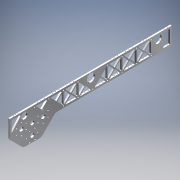
# Autodesk Inventor part: Inner Plate
Saved by Autodesk Inventor 2019.4 (Build 234330000, 330)
## iProperties
Created: 2019-12-07
Part Number: Inner Plate
Material: Aluminum 6061
Document SubType Name: Modeling
Designer: admin
Density: 2.7 g/cm^3
Appearance: Aluminum - Flat
Mass: 787.136 g
Surface Area: 1230.91 cm^2
Volume: 291.532 cm^3
Author: admin
Autodesk Inventor part; units mm, degrees
ref_plane "YZ Plane" through (0, 0, 0) normal (1, 0, 0) x (0, 1, 0)
sketch "Sketch1" plane through (0, 0, 0) normal (1, 0, 0) x (0, 1, 0)
  line L0 (80, -100) -> (0, -100)
  line L1 (0, -100) -> (0, 100)
  line L2 (0, 100) -> (80, 100)
  line L3 (80, 100) -> (80, -100)
  line L4 (30, -90) -> (30, 90) construction
  line L5 (30, 0) -> (95.4693, 0) construction
  line L6 (60, -40) -> (-60, -40) construction
  line L7 (-60, -40) -> (-60, 40)
  line L8 (-60, 40) -> (60, 40) construction
  line L9 (60, 40) -> (60, -40) construction
  line L10 (60, -40) -> (-60, 40) construction
  line L11 (-60, -40) -> (60, 40) construction
  line L12 (-60, -40) -> (0, -100)
  line L13 (-60, -40) -> (24.8528, -40) construction
  line L14 (-60, 40) -> (0, 100)
  point P0 (0, 0)
  point P1 (0, 0)
  point P2 (0, 0)
  dimension "d2" = 80
  dimension "d3" = 200
  dimension "d7" = 180
  dimension "d8" = 30
  dimension "d9" = 100
  dimension "d10" = 120
  dimension "d11" = 80
  dimension "d12" = 45
  dimension "d13" = 45
  constraints: 30 end point, 5 midpoint, 4 horizontal, 4 parallel, 2 perpendicular, 2 point on line, 1 coincident, 1 equal length, 1 vertical
  measures "d2" distance of L0.start L0.end
  measures "d3" distance of L2.end L0.start
  measures "d7" distance of L4.end L4.start
  measures "d8" distance between parallel lines of L1 L4
  measures "d9" distance between parallel lines of L0 L5
  measures "d10" distance of L7.end L8.end
  measures "d11" distance of L6.end L7.end
  measures "d12" angle of L12 L13
  measures "d13" angle of L8 L14
extrude "Extrusion1" add sketch "Sketch1" along normal blind 7
sketch "Sketch2" plane through (7, 0, 0) normal (1, 0, 0) x (0, 0, -1)
  circle A0 centre (0, 15.965) radius 9.5
  circle A1 centre (0, 15.965) radius 40.64 construction
  circle A2 centre (-48.26, 15.965) radius 7.62 construction
  circle A3 centre (0, -32.295) radius 7.62 construction
  circle A4 centre (48.26, 15.965) radius 7.62 construction
  line L0 (0, 0) -> (0, 40) construction
  line L1 (100, 80) -> (-100, 80) projected
  circle A5 centre (0, -32.295) radius 9.65
  circle A6 centre (-48.26, 15.965) radius 9.65
  circle A7 centre (48.26, 15.965) radius 9.65
  line L2 (0, 15.965) -> (-48.26, 15.965) construction
  line L3 (0, 15.965) -> (48.26, 15.965) construction
  circle A8 centre (0, -32.295) radius 25.4 construction
  circle A9 centre (12.7, -54.292) radius 2.75
  circle A10 centre (0, -32.295) radius 25.4 construction
  circle A11 centre (25.4, -32.295) radius 2.75
  circle A12 centre (0, -32.295) radius 25.4 construction
  circle A13 centre (12.7, -10.298) radius 2.75
  circle A14 centre (0, -32.295) radius 25.4 construction
  circle A15 centre (-12.7, -10.298) radius 2.75
  circle A16 centre (0, -32.295) radius 25.4 construction
  circle A17 centre (-25.4, -32.295) radius 2.75
  circle A18 centre (0, -32.295) radius 25.4 construction
  circle A19 centre (-12.7, -54.292) radius 2.75
  line L4 (0, -32.295) -> (0, -43.499)
  line L5 (0, -32.295) -> (-12.7, -54.292)
  circle A20 centre (48.26, 15.965) radius 25.4 construction
  circle A21 centre (48.26, -9.435) radius 2.75
  circle A22 centre (70.257, 3.265) radius 2.75
  circle A23 centre (70.257, 28.665) radius 2.75
  circle A24 centre (48.26, 41.365) radius 2.75
  circle A25 centre (26.263, 28.665) radius 2.75
  circle A26 centre (26.263, 3.265) radius 2.75
  line L6 (48.26, 15.965) -> (48.26, -34.035) construction
  line L7 (48.26, 15.965) -> (98.26, 15.965) construction
  circle A27 centre (-48.26, 15.965) radius 25.4 construction
  circle A28 centre (-48.26, -9.435) radius 2.75
  line L8 (-48.26, 15.965) -> (-48.26, -9.435)
  line L9 (-48.26, 15.965) -> (-22.86, 15.965) construction
  circle A29 centre (-26.263, 3.265) radius 2.75
  circle A30 centre (-26.263, 28.665) radius 2.75
  circle A31 centre (-48.26, 41.365) radius 2.75
  circle A32 centre (-70.257, 28.665) radius 2.75
  circle A33 centre (-70.257, 3.265) radius 2.75
  circle A34 centre (0, 15.965) radius 22.5 construction
  circle A35 centre (-35, 59.9998) radius 33.75 construction
  circle A36 centre (-35, 59.9998) radius 14
  circle A37 centre (-48.26, 15.965) radius 30 construction
  circle A38 centre (48.26, 15.965) radius 30 construction
  circle A39 centre (0, -32.295) radius 30 construction
  dimension "d28" = 50.8
  dimension "d36" = 50.8
  dimension "d44" = 50.8
  dimension "d14" = 19
  dimension "d15" = 81.28
  dimension "d16" = 15.24
  dimension "d17" = 15.24
  dimension "d18" = 15.24
  dimension "d20" = 64.035
  dimension "d21" = 19.3
  dimension "d22" = 19.3
  dimension "d23" = 19.3
  dimension "d24" = 90
  dimension "d25" = 90
  dimension "d29" = 5.5
  dimension "d32" = 360
  dimension "d35" = 30
  dimension "d37" = 5.5
  dimension "d40" = 360
  dimension "d42" = 50
  dimension "d43" = 90
  dimension "d45" = 5.5
  dimension "d46" = 90
  dimension "d49" = 360
  dimension "d52" = 45
  dimension "d53" = 67.5
  dimension "d54" = 35
  dimension "d55" = 28
  dimension "d68" = 60
  dimension "d69" = 60
  dimension "d70" = 60
  constraints: 32 centre point, 18 end point, 12 coincident, 4 tangent, 4 vertical, 3 point on line, 2 horizontal alignment, 2 perpendicular, 2 vertical alignment, 1 horizontal, 71 other
  measures "d14" diameter of A0
  measures "d15" diameter of A1
  measures "d16" diameter of A2
  measures "d17" diameter of A3
  measures "d18" diameter of A4
  measures "d20" distance from line of L1 A0.centre
  measures "d21" diameter of A5
  measures "d22" diameter of A6
  measures "d23" diameter of A7
  measures "d24" angle of L0 L2
  measures "d25" angle of L0 L3
  measures "d29" diameter of A9
  measures "d35" angle of L4 L5
  measures "d37" diameter of A21
  measures "d42" distance of L6.start L6.end
  measures "d43" angle of L6 L7
  measures "d45" diameter of A28
  measures "d46" angle of L8 L9
  measures "d52" diameter of A34
  measures "d53" diameter of A35
  measures "d54" distance from line of L0 A35.centre
  measures "d55" diameter of A36
  measures "d68" diameter of A37
  measures "d69" diameter of A38
  measures "d70" diameter of A39
extrude "Extrusion2" cut sketch "Sketch2" against normal blind 10
sketch "Sketch3" plane through (7, 0, 0) normal (1, 0, 0) x (0, 0, -1)
  line L0 (100, 80) -> (-100, 80) projected
  line L1 (100, 80) -> (620, 80)
  line L2 (620, 80) -> (620, 3)
  line L3 (620, 3) -> (100, 3)
  line L4 (100, 3) -> (100, 80)
  point P0 (0, 0)
  dimension "d56" = 520
  dimension "d57" = 77
  constraints: 8 end point, 2 parallel, 1 horizontal, 1 perpendicular
  measures "d56" distance of L2.end L3.end
  measures "d57" distance of L1.end L2.end
extrude "Extrusion3" add sketch "Sketch3" against normal blind 7
sketch "Sketch4" plane through (0, 0, 0) normal (-1, 0, 0) x (0, 0, 1)
  circle A0 centre (-557.002, 59) radius 18.5
  circle A1 centre (-261, 59) radius 18.5
  line L0 (-620, 80) -> (100, 80) projected
  line L1 (-620, 80) -> (-620, 3) projected
  line L2 (-620, 3) -> (-100, 3) projected
  line L3 (100, 80) -> (-620, 80) projected
  circle A2 centre (35, 59.9998) radius 14 projected
  point P0 (0, 0)
  point P1 (-100, 0)
  dimension "d60" = 37
  dimension "d61" = 37
  dimension "d62" = 21
  dimension "d64" = 21
  dimension "d71" = 296
  dimension "d72" = 296.002
  constraints: 2 centre point, 1 other
  measures "d60" diameter of A0
  measures "d61" diameter of A1
  measures "d62" distance from line of L0 A1.centre
  measures "d64" distance from line of L0 A0.centre
  measures "d71" horizontal distance of A2.centre A1.centre
  measures "d72" distance of A1.centre A0.centre
extrude "Extrusion4" cut sketch "Sketch4" against normal blind 7 contours A0 | A1
fillet "Fillet3" radius 20 5 edges at (3.5, 3, -100) (3.5, 0, -100) (3.5, -60, -40) (3.5, -60, 40) (3.5, 0, 100)
sketch "Sketch5" plane through (0, 0, 0) normal (-1, 0, 0) x (0, 0, 1)
  line L0 (-12.002, 71.5) -> (-72.002, 71.5) construction
  line L1 (-72.002, 71.5) -> (-72.002, 11.5) construction
  line L2 (-72.002, 11.5) -> (-12.002, 11.5) construction
  line L3 (-12.002, 11.5) -> (-12.002, 71.5) construction
  line L4 (-12.002, 71.5) -> (-72.002, 11.5) construction
  line L5 (-72.002, 71.5) -> (-12.002, 11.5) construction
  line L6 (-12.002, 15.0355) -> (-12.002, 67.9645)
  line L7 (-15.5375, 71.5) -> (-68.4665, 71.5)
  line L8 (-72.002, 67.9645) -> (-72.002, 15.0355)
  line L9 (-68.4665, 11.5) -> (-15.5375, 11.5)
  line L10 (-12.002, 15.0355) -> (-38.4665, 41.5)
  line L11 (-42.002, 45.0355) -> (-68.4665, 71.5)
  line L12 (-15.5375, 11.5) -> (-42.002, 37.9645)
  line L13 (-45.5375, 41.5) -> (-72.002, 67.9645)
  line L14 (-68.4665, 11.5) -> (-42.002, 37.9645)
  line L15 (-38.4665, 41.5) -> (-12.002, 67.9645)
  line L16 (-72.002, 15.0355) -> (-45.5375, 41.5)
  line L17 (-42.002, 45.0355) -> (-15.5375, 71.5)
  line L18 (-137.002, 15.0355) -> (-110.5375, 41.5)
  line L19 (-133.4665, 11.5) -> (-107.002, 37.9645)
  line L20 (-80.5375, 11.5) -> (-107.002, 37.9645)
  line L21 (-133.4665, 11.5) -> (-80.5375, 11.5)
  line L22 (-137.002, 67.9645) -> (-137.002, 15.0355)
  line L23 (-110.5375, 41.5) -> (-137.002, 67.9645)
  line L24 (-107.002, 45.0355) -> (-133.4665, 71.5)
  line L25 (-80.5375, 71.5) -> (-133.4665, 71.5)
  line L26 (-107.002, 45.0355) -> (-80.5375, 71.5)
  line L27 (-103.4665, 41.5) -> (-77.002, 67.9645)
  line L28 (-77.002, 11.5) -> (-77.002, 71.5) construction
  line L29 (-77.002, 15.0355) -> (-77.002, 67.9645)
  line L30 (-77.002, 15.0355) -> (-103.4665, 41.5)
  line L31 (-202.002, 15.0355) -> (-175.5375, 41.5)
  line L32 (-198.4665, 11.5) -> (-172.002, 37.9645)
  line L33 (-145.5375, 11.5) -> (-172.002, 37.9645)
  line L34 (-198.4665, 11.5) -> (-145.5375, 11.5)
  line L35 (-202.002, 67.9645) -> (-202.002, 15.0355)
  line L36 (-175.5375, 41.5) -> (-202.002, 67.9645)
  line L37 (-172.002, 45.0355) -> (-198.4665, 71.5)
  line L38 (-145.5375, 71.5) -> (-198.4665, 71.5)
  line L39 (-172.002, 45.0355) -> (-145.5375, 71.5)
  line L40 (-168.4665, 41.5) -> (-142.002, 67.9645)
  line L41 (-142.002, 11.5) -> (-142.002, 71.5) construction
  line L42 (-142.002, 15.0355) -> (-142.002, 67.9645)
  line L43 (-142.002, 15.0355) -> (-168.4665, 41.5)
  line L44 (-267.002, 15.0355) -> (-240.5375, 41.5)
  line L45 (-263.4665, 11.5) -> (-237.002, 37.9645)
  line L46 (-210.5375, 11.5) -> (-237.002, 37.9645)
  line L47 (-263.4665, 11.5) -> (-210.5375, 11.5)
  line L48 (-267.002, 67.9645) -> (-267.002, 15.0355)
  line L49 (-240.5375, 41.5) -> (-267.002, 67.9645)
  line L50 (-237.002, 45.0355) -> (-263.4665, 71.5)
  line L51 (-210.5375, 71.5) -> (-263.4665, 71.5)
  line L52 (-237.002, 45.0355) -> (-210.5375, 71.5)
  line L53 (-233.4665, 41.5) -> (-207.002, 67.9645)
  line L54 (-207.002, 11.5) -> (-207.002, 71.5) construction
  line L55 (-207.002, 15.0355) -> (-207.002, 67.9645)
  line L56 (-207.002, 15.0355) -> (-233.4665, 41.5)
  line L57 (-332.002, 15.0355) -> (-305.5375, 41.5)
  line L58 (-328.4665, 11.5) -> (-302.002, 37.9645)
  line L59 (-275.5375, 11.5) -> (-302.002, 37.9645)
  line L60 (-328.4665, 11.5) -> (-275.5375, 11.5)
  line L61 (-332.002, 67.9645) -> (-332.002, 15.0355)
  line L62 (-305.5375, 41.5) -> (-332.002, 67.9645)
  line L63 (-302.002, 45.0355) -> (-328.4665, 71.5)
  line L64 (-275.5375, 71.5) -> (-328.4665, 71.5)
  line L65 (-302.002, 45.0355) -> (-275.5375, 71.5)
  line L66 (-298.4665, 41.5) -> (-272.002, 67.9645)
  line L67 (-272.002, 11.5) -> (-272.002, 71.5) construction
  line L68 (-272.002, 15.0355) -> (-272.002, 67.9645)
  line L69 (-272.002, 15.0355) -> (-298.4665, 41.5)
  line L70 (-397.002, 15.0355) -> (-370.5375, 41.5)
  line L71 (-393.4665, 11.5) -> (-367.002, 37.9645)
  line L72 (-340.5375, 11.5) -> (-367.002, 37.9645)
  line L73 (-393.4665, 11.5) -> (-340.5375, 11.5)
  line L74 (-397.002, 67.9645) -> (-397.002, 15.0355)
  line L75 (-370.5375, 41.5) -> (-397.002, 67.9645)
  line L76 (-367.002, 45.0355) -> (-393.4665, 71.5)
  line L77 (-340.5375, 71.5) -> (-393.4665, 71.5)
  line L78 (-367.002, 45.0355) -> (-340.5375, 71.5)
  line L79 (-363.4665, 41.5) -> (-337.002, 67.9645)
  line L80 (-337.002, 11.5) -> (-337.002, 71.5) construction
  line L81 (-337.002, 15.0355) -> (-337.002, 67.9645)
  line L82 (-337.002, 15.0355) -> (-363.4665, 41.5)
  line L83 (-462.002, 15.0355) -> (-435.5375, 41.5)
  line L84 (-458.4665, 11.5) -> (-432.002, 37.9645)
  line L85 (-405.5375, 11.5) -> (-432.002, 37.9645)
  line L86 (-458.4665, 11.5) -> (-405.5375, 11.5)
  line L87 (-462.002, 67.9645) -> (-462.002, 15.0355)
  line L88 (-435.5375, 41.5) -> (-462.002, 67.9645)
  line L89 (-432.002, 45.0355) -> (-458.4665, 71.5)
  line L90 (-405.5375, 71.5) -> (-458.4665, 71.5)
  line L91 (-432.002, 45.0355) -> (-405.5375, 71.5)
  line L92 (-428.4665, 41.5) -> (-402.002, 67.9645)
  line L93 (-402.002, 11.5) -> (-402.002, 71.5) construction
  line L94 (-402.002, 15.0355) -> (-402.002, 67.9645)
  line L95 (-402.002, 15.0355) -> (-428.4665, 41.5)
  line L96 (-527.002, 15.0355) -> (-500.5375, 41.5)
  line L97 (-523.4665, 11.5) -> (-497.002, 37.9645)
  line L98 (-470.5375, 11.5) -> (-497.002, 37.9645)
  line L99 (-523.4665, 11.5) -> (-470.5375, 11.5)
  line L100 (-527.002, 67.9645) -> (-527.002, 15.0355)
  line L101 (-500.5375, 41.5) -> (-527.002, 67.9645)
  line L102 (-497.002, 45.0355) -> (-523.4665, 71.5)
  line L103 (-470.5375, 71.5) -> (-523.4665, 71.5)
  line L104 (-497.002, 45.0355) -> (-470.5375, 71.5)
  line L105 (-493.4665, 41.5) -> (-467.002, 67.9645)
  line L106 (-467.002, 11.5) -> (-467.002, 71.5) construction
  line L107 (-467.002, 15.0355) -> (-467.002, 67.9645)
  line L108 (-467.002, 15.0355) -> (-493.4665, 41.5)
  circle A0 centre (-74.502, 11.5) radius 2.75
  circle A1 centre (-74.502, 71.5) radius 2.75
  circle A2 centre (-139.502, 11.5) radius 2.75
  circle A3 centre (-139.502, 71.5) radius 2.75
  circle A4 centre (-204.502, 11.5) radius 2.75
  circle A5 centre (-204.502, 71.5) radius 2.75
  circle A6 centre (-269.502, 11.5) radius 2.75
  circle A7 centre (-269.502, 71.5) radius 2.75
  circle A8 centre (-334.502, 11.5) radius 2.75
  circle A9 centre (-334.502, 71.5) radius 2.75
  circle A10 centre (-399.502, 11.5) radius 2.75
  circle A11 centre (-399.502, 71.5) radius 2.75
  circle A12 centre (-464.502, 11.5) radius 2.75
  circle A13 centre (-464.502, 71.5) radius 2.75
  circle A14 centre (-529.502, 11.5) radius 2.75
  circle A15 centre (-529.502, 71.5) radius 2.75
  circle A16 centre (-9.502, 11.5) radius 2.75
  circle A17 centre (-9.502, 71.5) radius 2.75
  circle A18 centre (-74.502, 11.5) radius 2.75
  circle A19 centre (-74.502, 71.5) radius 2.75
  circle A20 centre (-139.502, 11.5) radius 2.75
  circle A21 centre (-139.502, 71.5) radius 2.75
  circle A22 centre (-204.502, 11.5) radius 2.75
  circle A23 centre (-204.502, 71.5) radius 2.75
  circle A24 centre (-269.502, 11.5) radius 2.75
  circle A25 centre (-269.502, 71.5) radius 2.75
  circle A26 centre (-334.502, 11.5) radius 2.75
  circle A27 centre (-334.502, 71.5) radius 2.75
  circle A28 centre (-399.502, 11.5) radius 2.75
  circle A29 centre (-399.502, 71.5) radius 2.75
  circle A30 centre (-464.502, 11.5) radius 2.75
  circle A31 centre (-464.502, 71.5) radius 2.75
  circle A32 centre (-557.002, 59) radius 18.5 projected
  line L109 (-620, 80) -> (100, 80) projected
  line L110 (-620, 3) -> (-111.2843, 3) projected
  line L111 (91.5, 21.5) -> (91.5, 71.5)
  line L112 (91.5, 71.5) -> (49.4831, 71.5)
  line L113 (49.4831, 71.5) -> (91.5, 21.5)
  line L114 (100, 80) -> (100, 8.2843) projected
  line L115 (-582.002, 71.5) -> (-582.002, 11.5)
  line L116 (-582.002, 11.5) -> (-611.5, 11.5)
  line L117 (-611.5, 11.5) -> (-611.5, 71.5)
  line L118 (-611.5, 71.5) -> (-582.002, 71.5)
  line L119 (-620, 80) -> (-620, 3) projected
  point P0 (0, 0)
  point P1 (-42.002, 41.5)
  point P2 (-555, 80)
  point P3 (35, 80)
  point P4 (-600, 3)
  dimension "d84" = 60
  dimension "d85" = 60
  dimension "d88" = 2.5
  dimension "d89" = 2.5
  dimension "d90" = 2.5
  dimension "d91" = 2.5
  dimension "d92" = 2.5
  dimension "d93" = 2.5
  dimension "d94" = 2.5
  dimension "d95" = 2.5
  dimension "d96" = 65
  dimension "d97" = 5.5
  dimension "d98" = 5.5
  dimension "d99" = 2.5
  dimension "d100" = 2.5
  dimension "d103" = 65
  dimension "d104" = 65
  dimension "d106" = 30
  dimension "d107" = 8.5
  dimension "d108" = 8.5
  dimension "d109" = 8.5
  dimension "d144" = 8.5
  dimension "d145" = 8.5
  dimension "d146" = 50
  dimension "d154" = 8.5
  dimension "d155" = 8.5
  dimension "d156" = 8.5
  dimension "d157" = 25
  constraints: 232 end point, 32 centre point, 22 point on line, 10 parallel, 5 perpendicular, 4 horizontal, 3 collinear, 2 midpoint, 2 vertical, 248 other
  measures "d84" distance of L2.end L1.end
  measures "d85" distance of L1.end L0.end
  measures "d88" distance between parallel lines of L4 L15
  measures "d89" distance between parallel lines of L4 L17
  measures "d90" distance between parallel lines of L5 L10
  measures "d91" distance between parallel lines of L5 L12
  measures "d92" distance between parallel lines of L4 L16
  measures "d93" distance between parallel lines of L4 L14
  measures "d94" distance between parallel lines of L5 L11
  measures "d95" distance between parallel lines of L5 L13
  measures "d96" distance of L8.end L18.start
  measures "d97" diameter of A0
  measures "d98" diameter of A1
  measures "d99" distance from line of L8 A1.centre
  measures "d100" distance from line of L8 A0.centre
  measures "d103" distance of A0.centre A2.centre
  measures "d104" distance of A0.centre A16.centre
  measures "d106" distance from line of A32.centre L100
  measures "d107" distance between parallel lines of L109 L103
  measures "d108" distance from line of L109 A11.centre
  measures "d109" distance from line of L110 A10.centre
  measures "d144" distance between parallel lines of L109 L112
  measures "d145" distance between parallel lines of L114 L111
  measures "d146" distance of L111.start L111.end
  measures "d154" distance between parallel lines of L110 L116
  measures "d155" distance between parallel lines of L109 L118
  measures "d156" distance between parallel lines of L119 L117
  measures "d157" distance from line of A32.centre L115
extrude "Extrusion5" cut sketch "Sketch5" against normal blind 10 contours L17 L11 L7 | L22 L23 L18 | L24 L25 L26 | L35 L36 L31 | L32 L33 L34 | L37 L38 L39 | L40 L42 L43 | L45 L46 L47 | L53 L55 L56 | L61 L62 L57 | L58 L59 L60 | L74 L75 L70 | L71 L72 L73 | L76 L77 L78 | L79 L81 L82 | L87 L88 L83 | L84 L85 L86 | L89 L90 L91 | L92 L94 L95 | L100 L101 L96 | L97 L98 L99 | L102 L103 L104 | L105 L107 L108 | A1 | A2 | A3 | A4 | A5 | A6 | A8 | A9 | A10 | A11 | A12 | A13 | A14 | A15 | A17 | L113 L112 L111 | L115 L116 L117 L118
sketch "Sketch6" plane through (0, 0, 0) normal (-1, 0, 0) x (0, 0, 1)
  circle A0 centre (-592.002, 11.5) radius 2.75
  line L0 (-527.002, 15.0355) -> (-527.002, 67.9645) projected
  line L1 (-620, 3) -> (-111.2843, 3) projected
  circle A1 centre (90, 11.5) radius 2.75
  line L2 (100, 80) -> (100, 8.2843) projected
  point P0 (0, 0)
  point P1 (-600, 3)
  point P2 (100, 15)
  dimension "d112" = 5.5
  dimension "d113" = 65
  dimension "d114" = 8.5
  dimension "d117" = 5.5
  dimension "d118" = 8.5
  dimension "d119" = 10
  constraints: 2 centre point
  measures "d112" diameter of A0
  measures "d113" distance from line of L0 A0.centre
  measures "d114" distance from line of L1 A0.centre
  measures "d117" diameter of A1
  measures "d118" distance from line of L1 A1.centre
  measures "d119" distance from line of L2 A1.centre
extrude "Extrusion6" [suppressed]
ref_plane "Work Plane2" through (7, 3, -600) normal (0, -1, 0) x (1, 0, 0)
sketch "Sketch7" plane through (7, 3, -600) normal (0, -1, 0) x (1, 0, 0)
  line L0 (0, 76.5335) -> (0, 129.4625) projected
  line L1 (-7, 76.5335) -> (0, 76.5335) projected
  line L2 (-7, 129.4625) -> (-7, 76.5335) projected
  line L3 (-7, 129.4625) -> (0, 129.4625) projected
  line L4 (0, 141.5335) -> (0, 194.4625) projected
  line L5 (-7, 141.5335) -> (0, 141.5335) projected
  line L6 (-7, 194.4625) -> (-7, 141.5335) projected
  line L7 (-7, 194.4625) -> (0, 194.4625) projected
  line L8 (0, 206.5335) -> (0, 259.4625) projected
  line L9 (-7, 206.5335) -> (0, 206.5335) projected
  line L10 (-7, 259.4625) -> (-7, 206.5335) projected
  line L11 (-7, 259.4625) -> (0, 259.4625) projected
  line L12 (0, 271.5335) -> (0, 324.4625) projected
  line L13 (-7, 271.5335) -> (0, 271.5335) projected
  line L14 (-7, 324.4625) -> (-7, 271.5335) projected
  line L15 (-7, 324.4625) -> (0, 324.4625) projected
  line L16 (0, 336.5335) -> (0, 389.4625) projected
  line L17 (-7, 336.5335) -> (0, 336.5335) projected
  line L18 (-7, 389.4625) -> (-7, 336.5335) projected
  line L19 (-7, 389.4625) -> (0, 389.4625) projected
  line L20 (0, 401.5335) -> (0, 454.4625) projected
  line L21 (-7, 401.5335) -> (0, 401.5335) projected
  line L22 (-7, 454.4625) -> (-7, 401.5335) projected
  line L23 (-7, 454.4625) -> (0, 454.4625) projected
  circle A0 centre (-3.5, 87.998) radius 1.65
  line L24 (-7, 102.998) -> (0, 102.998) projected
  circle A1 centre (-3.5, 102.998) radius 1.65
  circle A2 centre (-3.5, 117.998) radius 1.65
  line L25 (-3.5, 87.998) -> (-3.5, 117.998) construction
  circle A3 centre (-3.5, 152.998) radius 1.65
  circle A4 centre (-3.5, 167.998) radius 1.65
  circle A5 centre (-3.5, 182.998) radius 1.65
  circle A6 centre (-3.5, 217.998) radius 1.65
  circle A7 centre (-3.5, 232.998) radius 1.65
  circle A8 centre (-3.5, 247.998) radius 1.65
  circle A9 centre (-3.5, 282.998) radius 1.65
  circle A10 centre (-3.5, 297.998) radius 1.65
  circle A11 centre (-3.5, 312.998) radius 1.65
  circle A12 centre (-3.5, 347.998) radius 1.65
  circle A13 centre (-3.5, 362.998) radius 1.65
  circle A14 centre (-3.5, 377.998) radius 1.65
  circle A15 centre (-3.5, 412.998) radius 1.65
  circle A16 centre (-3.5, 427.998) radius 1.65
  circle A17 centre (-3.5, 442.998) radius 1.65
  point P0 (-7, 600)
  dimension "d120" = 3.3
  dimension "d121" = 3.3
  dimension "d122" = 3.3
  dimension "d123" = 15
  dimension "d124" = 15
  dimension "d125" = 15
  dimension "d128" = 65
  constraints: 18 centre point, 2 end point, 2 vertical, 1 midpoint, 30 other
  measures "d120" diameter of A0
  measures "d121" diameter of A1
  measures "d122" diameter of A2
  measures "d123" distance of A1.centre L25.start
  measures "d124" distance of L25.end A1.centre
  measures "d125" distance of L25.end A1.centre
  measures "d128" distance of L25.start A3.centre
extrude "Extrusion7" cut sketch "Sketch7" against normal up to surface (8.5 mm away) contours A1 L24 | L24 A1 | A0 | A2 | A3 | A4 | A5 | A6 | A7 | A8 | A9 | A10 | A11 | A12 | A13 | A14 | A15 | A16 | A17
ref_plane "Work Plane1" through (0, 80, 35) normal (0, 1, 0) x (1, 0, 0)
sketch "Sketch8" plane through (0, 80, 35) normal (0, 1, 0) x (1, 0, 0)
  circle A0 centre (3.5, 547.002) radius 1.65 projected
  circle A1 centre (3.5, 532.002) radius 1.65 projected
  circle A2 centre (3.5, 517.002) radius 1.65 projected
  circle A3 centre (3.5, 547.002) radius 1.65
  circle A4 centre (3.5, 532.002) radius 1.65
  circle A5 centre (3.5, 517.002) radius 1.65
  line L0 (7, 0) -> (7, 590) projected
  circle A6 centre (3.5, 482.002) radius 1.65
  circle A7 centre (3.5, 467.002) radius 1.65
  circle A8 centre (3.5, 452.002) radius 1.65
  circle A9 centre (3.5, 417.002) radius 1.65
  circle A10 centre (3.5, 402.002) radius 1.65
  circle A11 centre (3.5, 387.002) radius 1.65
  circle A12 centre (3.5, 352.002) radius 1.65
  circle A13 centre (3.5, 337.002) radius 1.65
  circle A14 centre (3.5, 322.002) radius 1.65
  circle A15 centre (3.5, 287.002) radius 1.65
  circle A16 centre (3.5, 272.002) radius 1.65
  circle A17 centre (3.5, 257.002) radius 1.65
  circle A18 centre (3.5, 222.002) radius 1.65
  circle A19 centre (3.5, 207.002) radius 1.65
  circle A20 centre (3.5, 192.002) radius 1.65
  circle A21 centre (3.5, 157.002) radius 1.65
  circle A22 centre (3.5, 142.002) radius 1.65
  circle A23 centre (3.5, 127.002) radius 1.65
  circle A24 centre (3.5, 92.002) radius 1.65
  circle A25 centre (3.5, 77.002) radius 1.65
  circle A26 centre (3.5, 62.002) radius 1.65
  point P0 (0, 35)
  dimension "d137" = 65
  constraints: 24 centre point, 3 coincident, 3 concentric, 1 vertical, 42 other
  measures "d137" distance of A3.centre A6.centre
extrude "Extrusion8" cut sketch "Sketch8" against normal up to surface (8.5 mm away) contours A0 | A1 | A2 | A6 | A7 | A8 | A9 | A10 | A11 | A18 | A19 | A20 | A21 | A22 | A23 | A24 | A25 | A26
sketch "Sketch9" plane through (0, 80, 100) normal (0, 1, 0) x (1, 0, 0)
  line L0 (7, 8.5) -> (7, 50.5169) projected
  line L1 (0, 8.5) -> (7, 8.5) projected
  line L2 (0, 50.5169) -> (0, 8.5) projected
  line L3 (0, 50.5169) -> (7, 50.5169) projected
  circle A0 centre (3.5, 29.5084) radius 1.65
  circle A1 centre (3.5, 19.5084) radius 1.65
  circle A2 centre (3.5, 39.5084) radius 1.65
  line L4 (3.5, 39.5084) -> (3.5, 29.5084) construction
  line L5 (3.5, 29.5084) -> (3.5, 19.5084) construction
  point P0 (0, 100)
  dimension "d147" = 3.3
  dimension "d148" = 3.3
  dimension "d149" = 3.3
  dimension "d150" = 10
  dimension "d151" = 10
  constraints: 4 end point, 3 centre point, 1 collinear, 1 vertical
  measures "d147" diameter of A0
  measures "d148" diameter of A1
  measures "d149" diameter of A2
  measures "d150" distance of L4.start L4.end
  measures "d151" distance of L4.end L5.end
extrude "Extrusion9" cut sketch "Sketch9" against normal up to surface (8.5 mm away) contours A0 | A1 | A2
sketch "Sketch10" plane through (0, 71.5, -611.5) normal (0, -1, 0) x (1, 0, 0)
  line L0 (7, 29.498) -> (7, 0) projected
  line L1 (0, 29.498) -> (7, 29.498) projected
  line L2 (0, 0) -> (0, 29.498) projected
  line L3 (0, 0) -> (7, 0) projected
  circle A0 centre (3.5, 7.5) radius 1.65
  circle A1 centre (3.5, 22.5) radius 1.65
  point P0 (0, 611.5)
  dimension "d158" = 3.3
  dimension "d159" = 3.3
  dimension "d160" = 15
  dimension "d161" = 3.5
  dimension "d162" = 3.5
  dimension "d163" = 7.5
  constraints: 2 centre point
  measures "d158" diameter of A0
  measures "d159" diameter of A1
  measures "d160" distance of A1.centre A0.centre
  measures "d161" distance from line of L2 A0.centre
  measures "d162" distance from line of L2 A1.centre
  measures "d163" distance from line of L3 A0.centre
extrude "Extrusion10" cut sketch "Sketch10" along normal through all both and the other way through all contours A0 | A1
fillet "Fillet5" radius 2 73 edges at (3.5, 67.9645, -527.002) (3.5, 71.5, -523.4665) (3.5, 15.0355, -527.002) (3.5, 11.5, -523.4665) (3.5, 11.5, -470.5375) (3.5, 15.0355, -467.002) (3.5, 67.9645, -467.002) (3.5, 71.5, -470.5375) (3.5, 37.9645, -497.002) (3.5, 41.5, -500.5375) (3.5, 45.0355, -497.002) (3.5, 41.5, -493.4665) (3.5, 37.9645, -432.002) (3.5, 41.5, -435.5375) (3.5, 41.5, -428.4665) (3.5, 45.0355, -432.002) (3.5, 11.5, -405.5375) (3.5, 11.5, -458.4665) (3.5, 67.9645, -462.002) (3.5, 71.5, -458.4665) (3.5, 71.5, -405.5375) (3.5, 67.9645, -402.002) (3.5, 15.0355, -402.002) (3.5, 71.5, -340.5375) (3.5, 67.9645, -397.002) (3.5, 15.0355, -397.002) (3.5, 11.5, -393.4665) (3.5, 11.5, -340.5375) (3.5, 15.0355, -337.002) (3.5, 15.0355, -332.002) (3.5, 37.9645, -367.002) (3.5, 41.5, -370.5375) (3.5, 41.5, -363.4665) (3.5, 45.0355, -367.002) (3.5, 67.9645, -337.002) (3.5, 11.5, -328.4665) (3.5, 37.9645, -302.002) (3.5, 11.5, -275.5375) (3.5, 67.9645, -332.002) (3.5, 41.5, -305.5375) (3.5, 11.5, -263.4665) (3.5, 37.9645, -237.002) (3.5, 11.5, -210.5375) (3.5, 67.9645, -207.002) (3.5, 41.5, -233.4665) (3.5, 15.0355, -207.002) (3.5, 15.0355, -202.002) (3.5, 67.9645, -202.002) (3.5, 41.5, -175.5375) (3.5, 37.9645, -172.002) (3.5, 11.5, -198.4665) (3.5, 11.5, -145.5375) (3.5, 41.5, -168.4665) (3.5, 67.9645, -142.002) (3.5, 71.5, -145.5375) (3.5, 71.5, -198.4665) (3.5, 45.0355, -172.002) (3.5, 67.9645, -137.002) (3.5, 15.0355, -137.002) (3.5, 41.5, -110.5375) (3.5, 45.0355, -107.002) (3.5, 71.5, -133.4665) (3.5, 71.5, -80.5375) (3.5, 71.5, -68.4665) (3.5, 45.0355, -42.002) (3.5, 71.5, -15.5375) (3.5, 71.5, 49.4831) (3.5, 71.5, 91.5) (3.5, 21.5, 91.5) (3.5, 71.5, -582.002) (3.5, 71.5, -611.5) (3.5, 11.5, -611.5) (3.5, 11.5, -582.002)
equation "\"d9\" = 0.5 * d3"
body "Solid1"
